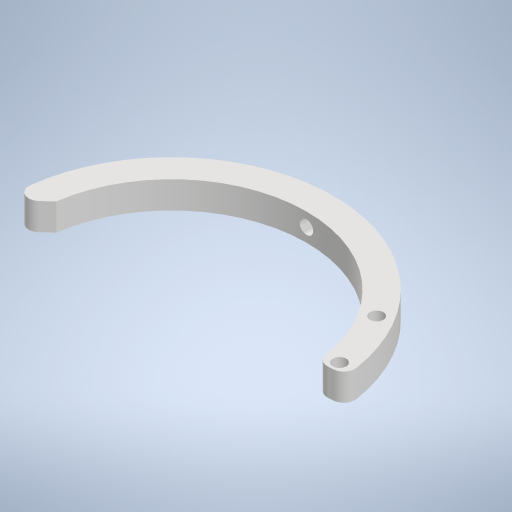
# Autodesk Inventor part: ganascia
Saved by Autodesk Inventor 2023 (Build 270158000, 158)
## iProperties
Created: 2023-08-01
Part Number: ganascia
Material: Generico
Document SubType Name: Modeling
Designer: Admin
Density: 1 g/cm^3
Appearance: Default
Author: Admin
Autodesk Inventor part; units mm, degrees
ref_plane "YZ Plane" through (0, 0, 0) normal (1, 0, 0) x (0, 1, 0)
ref_plane "XZ Plane" through (0, 0, 0) normal (0, 1, 0) x (-1, 0, 0)
ref_plane "XY Plane" through (0, 0, 0) normal (0, 0, 1) x (1, 0, 0)
sketch "Schizzo1" plane through (0, 0, 0) normal (0, 1, 0) x (-1, 0, 0)
  arc A0 (-49.8426, -3.9646) -> (50, 0) centre (0, 0) ccw
  arc A1 (-59.8111, -4.7575) -> (60, 0) centre (0, 0) ccw
  line L0 (60, 0) -> (50, 0)
  circle A2 centre (-54.4546, -7.7263) radius 2.5
  line L1 (-49.8426, -3.9646) -> (-59.8111, -4.7575)
  dimension "d0" = 100
  dimension "d6" = 5
  dimension "d8" = 2.5
  dimension "d9" = 2.5
  constraints: 4 end point, 4 point on circle, 3 centre point, 3 line through centre, 1 coincident, 1 horizontal
  measures "d0" diameter of A0
  measures "d6" diameter of A2
extrude "Estrusione1" add sketch "Schizzo1" along normal mid plane 10 contours A0 L0 A1 L1 | A2
extrude "Estrusione2" cut sketch "Schizzo1" along normal through all both and the other way through all contours A2
fillet "Raccordo3" radius 4 1 edges at (59.8111, 0, -4.7575)
fillet "Raccordo4" radius 4 1 edges at (49.8426, 0, -3.9646)
chamfer "Smusso1" distance 7 angle 45 1 edges at (-50, 0, 0)
fillet "Raccordo5" radius 4 2 edges at (-60, 0, 0) (-57, 0, 0)
sketch "Schizzo2" plane through (0, 5, 0) normal (0, 1, 0) x (1, 0, 0)
  circle A0 centre (46.4198, 29.499) radius 2.5
  circle A1 centre (54.4546, 7.7263) radius 2.5 projected
  arc A2 (49.412, 7.6457) -> (-49.51, 6.9828) centre (0, 0) ccw projected
  line L0 (42.1413, 26.9094) -> (50.6984, 32.0886) construction
  arc A3 (59.3185, 9.0175) -> (-59.5579, 7.2704) centre (0, 0) ccw projected
  dimension "d19" = 29.499
  dimension "d20" = 24.2008
  constraints: 2 end point, 2 point on circle, 1 centre point, 1 equal radius, 1 midpoint
  measures "d19" vertical distance of A2.centre A0.centre
  measures "d20" distance from line of A3.start L0
extrude "Estrusione3" cut sketch "Schizzo2" against normal blind 10 contours A0
sketch "Schizzo4" plane through (0, 0, 0) normal (0, 0, 1) x (1, 0, 0)
  circle A0 centre (0, 0) radius 2.5
  dimension "d28" = 5
  constraints: 1 centre point, 1 coincident
  measures "d28" diameter of A0
extrude "Estrusione5" cut sketch "Schizzo4" against normal through all
